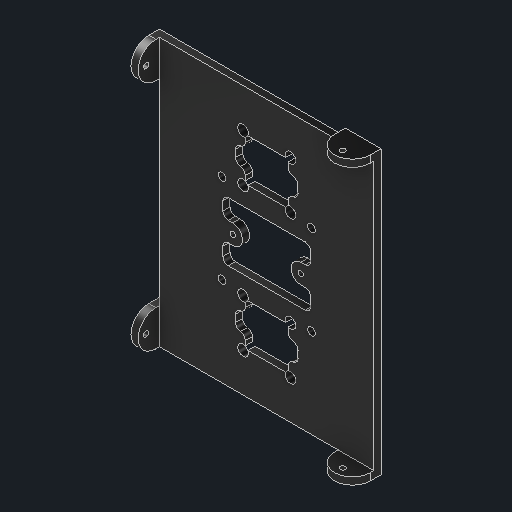
# Autodesk Inventor part: LED_mount
Saved by Autodesk Inventor 2026.1 (Build 301233000, 233)
## iProperties
Created: 2026-01-20
Part Number: LED_mount
Material: ABS Plastic
Document SubType Name: Modeling
Designer: aleja
Density: 1.06 g/cm^3
Appearance: Glossy - Black
Author: aleja
Autodesk Inventor part; units mm, degrees
ref_plane "YZ Plane" through (0, 0, 0) normal (1, 0, 0) x (0, 1, 0)
ref_plane "XZ Plane" through (0, 0, 0) normal (0, 1, 0) x (-1, 0, 0)
ref_plane "XY Plane" through (0, 0, 0) normal (0, 0, 1) x (1, 0, 0)
sketch "Sketch1" plane through (0, 0, 0) normal (0, 1, 0) x (-1, 0, 0)
  line L0 (-60, 75) -> (60, 75)
  line L1 (60, 75) -> (60, -75)
  line L2 (60, -75) -> (-60, -75)
  line L3 (-60, -75) -> (-60, 75)
  line L4 (-60, 75) -> (60, -75) construction
  line L5 (60, 75) -> (-60, -75) construction
  point P0 (0, 0)
  dimension "d0" = 120
  dimension "d1" = 150
  constraints: 12 end point, 2 midpoint, 2 parallel, 1 horizontal, 1 perpendicular
  measures "d0" distance of L1.end L2.end
  measures "d1" distance of L0.end L1.end
extrude "Extrusion1" add sketch "Sketch1" along normal blind 4
sketch "Sketch2" plane through (0, 4, 0) normal (0, 1, 0) x (1, 0, 0)
  line L0 (24.55, -16.5) -> (-24.55, -16.5)
  line L1 (-24.55, -16.5) -> (-24.55, 16.5)
  line L2 (-24.55, 16.5) -> (24.55, 16.5)
  line L3 (24.55, 16.5) -> (24.55, -16.5)
  line L4 (24.55, -16.5) -> (-24.55, 16.5) construction
  line L5 (-24.55, -16.5) -> (24.55, 16.5) construction
  line L6 (-24.55, 0) -> (-19.05, 0) construction
  arc A0 (-19.05, -5.5) -> (-19.05, 5.5) centre (-19.05, 0) ccw
  circle A1 centre (-19.05, 0) radius 1.5
  line L7 (-24.55, -5.5) -> (-19.05, -5.5)
  line L8 (-19.05, 5.5) -> (-24.55, 5.5)
  line L9 (0, 0) -> (0, 7.865527) construction
  arc A2 (19.05, 5.5) -> (19.05, -5.5) centre (19.05, 0) ccw
  circle A3 centre (19.05, 0) radius 1.5
  line L10 (24.55, -5.5) -> (19.05, -5.5)
  line L11 (19.05, 5.5) -> (24.55, 5.5)
  line L12 (10.522822, -52) -> (-10.522822, -52)
  line L13 (-12, -50.522822) -> (-12, -29.477178)
  line L14 (-10.522822, -28) -> (10.522822, -28)
  line L15 (12, -29.477178) -> (12, -50.522822)
  line L16 (12, -52) -> (-12, -28) construction
  line L17 (-12, -52) -> (12, -28) construction
  line L18 (13.25, -53.25) -> (-13.25, -53.25) construction
  line L19 (-13.25, -53.25) -> (-13.25, -26.75) construction
  line L20 (-13.25, -26.75) -> (13.25, -26.75) construction
  line L21 (13.25, -26.75) -> (13.25, -53.25) construction
  line L22 (13.25, -53.25) -> (-13.25, -26.75) construction
  line L23 (-13.25, -53.25) -> (13.25, -26.75) construction
  arc A4 (-12, -50.522822) -> (-10.522822, -52) centre (-13.25, -53.25) ccw
  arc A5 (-10.522822, -28) -> (-12, -29.477178) centre (-13.25, -26.75) ccw
  arc A6 (10.522822, -52) -> (12, -50.522822) centre (13.25, -53.25) ccw
  arc A7 (12, -29.477178) -> (10.522822, -28) centre (13.25, -26.75) ccw
  line L24 (17.5, -45) -> (-17.5, -45)
  line L25 (-17.5, -45) -> (-17.5, -35)
  line L26 (-17.5, -35) -> (17.5, -35)
  line L27 (17.5, -35) -> (17.5, -45)
  line L28 (17.5, -45) -> (-17.5, -35) construction
  line L29 (-17.5, -45) -> (17.5, -35) construction
  line L30 (10.522822, 52) -> (-10.522822, 52)
  line L31 (-12, 50.522822) -> (-12, 29.477178)
  line L32 (-10.522822, 28) -> (10.522822, 28)
  line L33 (12, 29.477178) -> (12, 50.522822)
  line L34 (12, 52) -> (-12, 28) construction
  line L35 (-12, 52) -> (12, 28) construction
  line L36 (13.25, 53.25) -> (-13.25, 53.25) construction
  line L37 (-13.25, 53.25) -> (-13.25, 26.75) construction
  line L38 (-13.25, 26.75) -> (13.25, 26.75) construction
  line L39 (13.25, 26.75) -> (13.25, 53.25) construction
  line L40 (13.25, 53.25) -> (-13.25, 26.75) construction
  line L41 (-13.25, 53.25) -> (13.25, 26.75) construction
  arc A8 (-10.522822, 52) -> (-12, 50.522822) centre (-13.25, 53.25) ccw
  arc A9 (-12, 29.477178) -> (-10.522822, 28) centre (-13.25, 26.75) ccw
  arc A10 (12, 50.522822) -> (10.522822, 52) centre (13.25, 53.25) ccw
  arc A11 (10.522822, 28) -> (12, 29.477178) centre (13.25, 26.75) ccw
  line L42 (17.5, 45) -> (-17.5, 45)
  line L43 (-17.5, 45) -> (-17.5, 35)
  line L44 (-17.5, 35) -> (17.5, 35)
  line L45 (17.5, 35) -> (17.5, 45)
  line L46 (17.5, 45) -> (-17.5, 35) construction
  line L47 (-17.5, 45) -> (17.5, 35) construction
  point P0 (0, 0)
  point P1 (0, -40)
  point P2 (0, 40)
  point P3 (-12, 45)
  point P4 (-12, 35)
  point P5 (12, -45)
  point P6 (12, -35)
  point P7 (-12, -35)
  point P8 (-12, -45)
  point P9 (12, 45)
  point P10 (12, 35)
  dimension "d4" = 49.1
  dimension "d5" = 33
  dimension "d6" = 5.5
  dimension "d7" = 3
  dimension "d8" = 24
  dimension "d9" = 24
  dimension "d10" = 40
  dimension "d11" = 26.5
  dimension "d12" = 26.5
  dimension "d13" = 6
  dimension "d14" = 6
  dimension "d15" = 6
  dimension "d16" = 6
  dimension "d17" = 35
  dimension "d18" = 10
  dimension "d64" = 5.5
  constraints: 96 end point, 31 symmetric about line, 20 point on circle, 12 centre point, 10 midpoint, 10 parallel, 9 coincident, 5 horizontal, 5 perpendicular, 2 point on line, 1 tangent, 1 vertical, 6 other
  measures "d4" distance of L1.end L2.end
  measures "d5" distance of L0.end L1.end
  measures "d6" distance of L6.start L6.end
  measures "d7" diameter of A1
  measures "d8" distance of L16.end L17.end
  measures "d9" distance of L17.start L16.end
  measures "d10" distance of point (0, 0) point (0, -40)
  measures "d11" distance of L19.end L20.end
  measures "d12" distance of L18.end L19.end
  measures "d13" diameter of A4
  measures "d14" diameter of A5
  measures "d15" diameter of A6
  measures "d16" diameter of A7
  measures "d17" distance of L25.end L26.end
  measures "d18" distance of L24.end L25.end
  measures "d64" radius of A0
extrude "Extrusion2" cut sketch "Sketch2" against normal through all contours L0 L1 L7 A0 L8 L2 L3 L11 A2 L10 | A1 | A3 | L12 A4 L13 L24 L15 A6 | L24 L13 L26 L15 | L15 L26 L27 L24 | L24 L25 L26 L13 | L26 L13 A5 L14 A7 L15 | A10 L33 L42 L31 A8 L30 | L42 L45 L44 L33 | L33 L44 L31 L42 | L31 L44 L43 L42 | L33 A11 L32 A9 L31 L44
sketch "Sketch3" plane through (0, 0, 0) normal (0, -1, 0) x (1, 0, 0)
  line L0 (-60, 75) -> (60, 75)
  line L1 (-60, 75) -> (-64, 75)
  line L2 (-64, 75) -> (-64, 55)
  line L3 (-64, 55) -> (-60, 55)
  line L4 (-60, 55) -> (-60, 75)
  line L5 (-64, 75) -> (-40, 75)
  line L6 (-40, 75) -> (-40, 79)
  line L7 (-40, 79) -> (-64, 79)
  line L8 (-64, 79) -> (-64, 75)
  line L9 (-60, -75) -> (-60, 75)
  line L10 (-60, 0) -> (-43.506886, 0) construction
  line L11 (-60, -75) -> (-64, -75)
  line L12 (-64, -75) -> (-64, -55)
  line L13 (-64, -55) -> (-60, -55)
  line L14 (-60, -55) -> (-60, -75)
  line L15 (-64, -75) -> (-40, -75)
  line L16 (-40, -75) -> (-40, -79)
  line L17 (-40, -79) -> (-64, -79)
  line L18 (-64, -79) -> (-64, -75)
  line L19 (0, 75) -> (0, 63.1817) construction
  line L20 (60, 75) -> (64, 75)
  line L21 (64, 75) -> (64, 55)
  line L22 (64, 55) -> (60, 55)
  line L23 (60, 55) -> (60, 75)
  line L24 (64, 75) -> (40, 75)
  line L25 (40, 75) -> (40, 79)
  line L26 (40, 79) -> (64, 79)
  line L27 (64, 79) -> (64, 75)
  line L28 (60, -75) -> (60, 75)
  line L29 (60, 0) -> (43.506886, 0) construction
  line L30 (60, -75) -> (64, -75)
  line L31 (64, -75) -> (64, -55)
  line L32 (64, -55) -> (60, -55)
  line L33 (60, -55) -> (60, -75)
  line L34 (64, -75) -> (40, -75)
  line L35 (40, -75) -> (40, -79)
  line L36 (40, -79) -> (64, -79)
  line L37 (64, -79) -> (64, -75)
  line L38 (60, -75) -> (60, -79)
  line L39 (60, 75) -> (60, 79)
  point P0 (0, 0)
  dimension "d21" = 4
  dimension "d22" = 20
  dimension "d23" = 24
  dimension "d24" = 4
  constraints: 76 end point, 21 symmetric about line, 4 parallel, 3 horizontal, 3 perpendicular, 3 point on line, 2 midpoint, 1 vertical
  measures "d21" distance of L3.end L2.end
  measures "d22" distance of L2.end L1.end
  measures "d23" distance of L7.end L6.end
  measures "d24" distance of L6.end L5.end
extrude "Extrusion3" add sketch "Sketch3" along normal blind 15 and the other way blind 4 contours L4 L3 L2 L1 | L25 L26 L39 L0 | L11 L12 L13 L9 | L38 L36 L35 L34
fillet "Fillet1" radius 3 24 edges at (24.55, 2, -16.5) (24.55, 2, -5.5) (24.55, 2, 16.5) (24.55, 2, 5.5) (-24.55, 2, -16.5) (-24.55, 2, -5.5) (-24.55, 2, 5.5) (-24.55, 2, 16.5) (-12, 2, -45) (-17.5, 2, -45) (12, 2, -35) (17.5, 2, -35) (12, 2, 45) (17.5, 2, 45) (-12, 2, 45) (-17.5, 2, 45) (-12, 2, 35) (-17.5, 2, 35) (-17.5, 2, -35) (-12, 2, -35) (17.5, 2, -45) (12, 2, -45) (17.5, 2, 35) (12, 2, 35)
sketch "Sketch7" plane through (-60, 0, -55) normal (1, 0, 0) x (0, 0, -1)
  line L0 (0, -15) -> (20, -15)
  line L1 (10, -15) -> (10, 0)
  line L2 (20, 0) -> (0, 0)
  circle A0 centre (10, -7.5) radius 1.5
  line L3 (-55, 0) -> (-55, -12.305526)
  circle A1 centre (-120, -7.5) radius 1.5
  dimension "d47" = 3
  constraints: 4 end point, 3 midpoint, 2 centre point, 1 symmetric about line, 1 vertical, 1 other
  measures "d47" diameter of A0
extrude "Extrusion8" cut sketch "Sketch7" against normal through all
sketch "Sketch8" plane through (60, 0, 75) normal (0, 0, -1) x (-1, 0, 0)
  line L0 (20, -15) -> (0, -15) projected
  line L1 (10, -15) -> (10, 0)
  line L2 (20, 0) -> (0, 0) projected
  circle A0 centre (10, -7.5) radius 1.5
  point P0 (60, 0)
  dimension "d50" = 3
  constraints: 3 midpoint, 2 end point, 1 centre point
  measures "d50" diameter of A0
extrude "Extrusion9" cut sketch "Sketch8" along normal through all both and the other way through all
sketch "Sketch9" plane through (0, -15, 0) normal (0, -1, 0) x (1, 0, 0)
  line L0 (-64, -55) -> (-64, -75) projected
  line L1 (-60, -75) -> (-60, -55) projected
  line L2 (-60, -55) -> (-64, -55) projected
  line L3 (-64, -75) -> (-60, -75) projected
  line L4 (-64, 55) -> (-60, 55) projected
  line L5 (-60, 55) -> (-60, 75) projected
  line L6 (-60, 75) -> (-64, 75) projected
  line L7 (-64, 75) -> (-64, 55) projected
  line L8 (60, 79) -> (40, 79) projected
  line L9 (40, 79) -> (40, 75) projected
  line L10 (40, 75) -> (60, 75) projected
  line L11 (60, 75) -> (60, 79) projected
  line L12 (40, -79) -> (60, -79) projected
  line L13 (60, -79) -> (60, -75) projected
  line L14 (60, -75) -> (40, -75) projected
  line L15 (40, -75) -> (40, -79) projected
  point P0 (0, 0)
extrude "Extrusion10" cut sketch "Sketch9" against normal blind 3
fillet "Fillet2" radius 10 8 edges at (-62, -12, -55) (-62, -12, -75) (-62, -12, 55) (-62, -12, 75) (40, -12, 77) (60, -12, 77) (60, -12, -77) (40, -12, -77)
sketch "Sketch10" plane through (0, 4, 0) normal (0, 1, 0) x (1, 0, 0)
  line L0 (25, 25) -> (-25, 25) construction
  line L1 (-25, 25) -> (-25, -25) construction
  line L2 (-25, -25) -> (25, -25) construction
  line L3 (25, -25) -> (25, 25) construction
  line L4 (25, 25) -> (-25, -25) construction
  line L5 (-25, 25) -> (25, -25) construction
  circle A0 centre (25, -25) radius 2.15
  circle A1 centre (-25, -25) radius 2.15
  circle A2 centre (-25, 25) radius 2.15
  circle A3 centre (25, 25) radius 2.15
  point P0 (0, 0)
  dimension "d56" = 50
  dimension "d57" = 50
  dimension "d58" = 4.3
  dimension "d59" = 4.3
  dimension "d60" = 4.3
  dimension "d61" = 4.3
  constraints: 12 end point, 4 centre point, 4 coincident, 2 midpoint, 2 parallel, 1 horizontal, 1 perpendicular
  measures "d56" distance of L1.end L2.end
  measures "d57" distance of L0.end L1.end
  measures "d58" diameter of A0
  measures "d59" diameter of A1
  measures "d60" diameter of A2
  measures "d61" diameter of A3
extrude "Extrusion11" cut sketch "Sketch10" against normal through all
body "Solid1"
